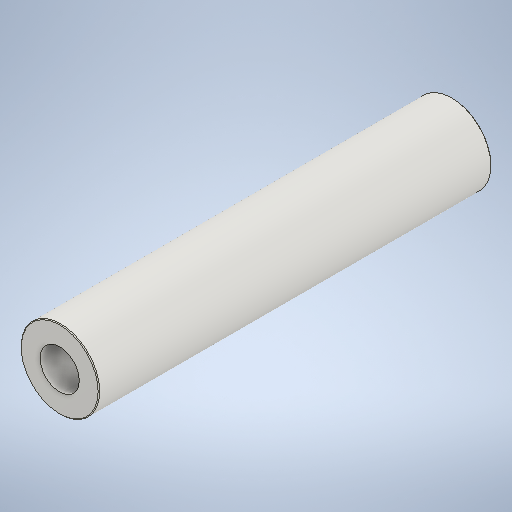
# Autodesk Inventor part: 34 - Base Pillar
Saved by Autodesk Inventor 2025.2 (Build 292293000, 293)
## iProperties
Created: 2025-07-30
Part Number: 34 - Base Pillar
Material: Steel AISI 1020 107 HR
Document SubType Name: Modeling
Designer: bless
Density: 7.87 g/cm^3
Appearance: Steel
Author: bless
Autodesk Inventor part; units mm, degrees
ref_plane "YZ Plane" through (0, 0, 0) normal (1, 0, 0) x (0, 1, 0)
ref_plane "XZ Plane" through (0, 0, 0) normal (0, 1, 0) x (-1, 0, 0)
ref_plane "XY Plane" through (0, 0, 0) normal (0, 0, 1) x (1, 0, 0)
sketch "Sketch1" plane through (0, 0, 0) normal (0, 0, 1) x (1, 0, 0)
  circle A0 centre (0, 0) radius 5
  circle A1 centre (0, 0) radius 2.5
  dimension "d0" = 10
  dimension "d1" = 5
  constraints: 2 centre point, 2 coincident
  measures "d0" diameter of A0
  measures "d1" diameter of A1
extrude "Extrusion1" add sketch "Sketch1" against normal blind 50
chamfer "Chamfer1" distance 0.1 angle 45 2 edges at (-5, 0, 0) (-5, 0, -50)
body "Solid1"
